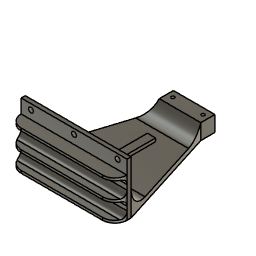
Adaptador (Autodesk Fusion 360 design; units mm, degrees)
Autodesk Fusion 360 part; units mm, degrees
sketch "Esboço1" plane through (0, 0, 0) normal (0, 0, 1) x (1, 0, 0)
  line L0 (0, 0) -> (65, 0)
  line L1 (0, 0) -> (-65, 0)
  line L2 (-65, 0) -> (-65, 5)
  line L3 (65, 0) -> (65, 5)
  line L4 (-65, 5) -> (65, 5)
  constraint coincident L0.start L1.start
  constraint horizontal L0
  constraint parallel L0 L1
  constraint perpendicular L1 L2
  constraint perpendicular L0 L3
  constraint perpendicular L3 L4
extrude "Extrusão1" add sketch "Esboço1" along normal blind 65 makes body 1
sketch "Esboço2" plane through (0, 0, 0) normal (0, 1, 0) x (1, 0, 0)
  line L0 (-65, 0) -> (-65, -15)
  line L1 (-65, -15) -> (65, -15)
  line L2 (65, -15) -> (65, 0)
  dimension "d7" = 15
  constraint vertical L0
  constraint perpendicular L0 L1
  constraint perpendicular L1 L2
  measures "d7" distance of L0.start L0.end
sketch "Esboço3" plane through (0, 0, 0) normal (0, 0, 1) x (1, 0, 0)
  line L0 (0.0189, 130) -> (-25.4811, 130)
  line L1 (0.0189, 130) -> (25.5189, 130)
  line L2 (-25.4811, 130) -> (-65, 5)
  line L3 (25.5189, 130) -> (65, 5)
  line L4 (65, 5) -> (-65, 5)
  line L5 (0, 0) -> (0, 130)
  dimension "d68" = 130
  constraint horizontal L4
  constraint coincident L5.start origin
  constraint perpendicular L4 L5
  measures "d68" distance of L5.start L5.end
extrude "Extrusão2" add sketch "Esboço3" along normal blind 6 bodies 1
sketch "Esboço4" plane through (0, 0, 0) normal (0, 0, 1) x (1, 0, 0)
  line L0 (-25.4811, 130) -> (-25.4811, 137.353)
  line L1 (25.5189, 130) -> (25.5189, 137.353)
  line L2 (25.5189, 137.353) -> (-25.4811, 137.353)
  line L3 (-25.4811, 130) -> (25.5189, 130)
  point P0 (25.5189, 130)
  constraint vertical L0
  constraint vertical L1
  constraint perpendicular L1 L2
  constraint coincident P0 L1.start
extrude "Extrusão4" add sketch "Esboço4" against normal blind 9 separate body makes body 2
extrude "Extrusão5" add sketch "Esboço4" along normal blind 6 bodies 1 2
sketch "Esboço5" plane through (0, 0, 0) normal (0, 0, 1) x (1, 0, 0)
  line L0 (0, 15) -> (-5, 15)
  line L1 (0, 15) -> (5, 15)
  line L2 (5, 15) -> (5, 95)
  line L3 (5, 95) -> (-5, 95)
  line L4 (-5, 95) -> (-5, 15)
  constraint horizontal L0
  constraint parallel L0 L1
  constraint perpendicular L1 L2
  constraint perpendicular L2 L3
  constraint perpendicular L0 L4
extrude "Extrusão6" add sketch "Esboço5" along normal blind 10 bodies 1
sketch "Esboço6" plane through (0, 0, 0) normal (0, 1, 0) x (1, 0, 0)
extrude "Extrusão7" add 1 faces at (-8.4811, 132.451, -9) along direction (0, 0, -1) blind 7 on bodies 1 bodies 1
extrude "Extrusão8" add 1 faces at (-8.4811, 137.353, -8.6667) along direction (0, 1, 0) blind 10 on bodies 1 bodies 1
sketch "Esboço7" plane through (0, 0, 0) normal (0, -1, 0) x (1, 0, 0)
  line L0 (-65, 0) -> (65, 0)
  line L1 (65, 0) -> (65, 65)
  line L2 (65, 65) -> (-65, 65)
  line L3 (-65, 65) -> (-65, 0)
  line L4 (-65, 48) -> (65, 48)
  line L5 (-65, 48) -> (65, 48)
  line L6 (65, 48) -> (65, 45)
  line L7 (65, 45) -> (-65, 45)
  line L8 (-65, 45) -> (-65, 48)
  line L9 (-65, 25) -> (65, 25)
  line L10 (65, 25) -> (65, 22)
  line L11 (65, 22) -> (-65, 22)
  line L12 (-65, 22) -> (-65, 25)
  line L13 (-65, 0) -> (65, 0)
  line L14 (65, 0) -> (65, 3)
  line L15 (65, 3) -> (-65, 3)
  line L16 (-65, 3) -> (-65, 0)
  dimension "d69" = 17
  dimension "d70" = 3
  dimension "d71" = 3
  dimension "d72" = 3
  dimension "d75" = 19
  constraint coincident L3 L4.start
  constraint coincident L1 L4.end
  constraint perpendicular L1 L4
  constraint horizontal L5
  constraint vertical L6
  constraint horizontal L7
  constraint vertical L8
  constraint horizontal L9
  constraint vertical L10
  constraint horizontal L11
  constraint vertical L12
  constraint coincident L3 L9.start
  constraint horizontal L13
  constraint vertical L14
  constraint horizontal L15
  constraint vertical L16
  constraint coincident L0.start L3.end
  measures "d69" distance of L2 L4
  measures "d70" distance of L4.start L7.end
  measures "d71" distance of L9.start L11.end
  measures "d72" distance of L0.start L15.end
  measures "d75" distance of L11 L15
hole "Furo6" at (-0.0241, 0, 58.8054) direction (0, 1, 0) diameter 6 depth 30 tip angle 118 bodies 1
hole "Furo7" at (-52.9048, 0, 58.2429) direction (0, 1, 0) diameter 6 depth 30 tip angle 118 bodies 1
hole "Furo8" at (53.4557, 0, 59.0312) direction (0, 1, 0) diameter 6 depth 30 tip angle 118 bodies 1
sketch "Esboço8" plane through (0, 0, 6) normal (0, 0, 1) x (-1, 0, 0)
  line L0 (-25.5189, -130) -> (-25.5189, -147.353)
  line L1 (-25.5189, -147.353) -> (25.4811, -147.353)
  line L2 (25.4811, -147.353) -> (25.4811, -130)
  line L3 (25.4811, -130) -> (-25.5189, -130)
  line L4 (-25.5189, -147.353) -> (25.4811, -147.353)
  line L5 (5, -15) -> (5, -95)
  line L6 (5, -95) -> (-5, -95)
  line L7 (-5, -95) -> (-5, -15)
  line L8 (-5, -15) -> (5, -15)
  line L9 (25.4811, -130) -> (65, -5)
  line L10 (65, -5) -> (-65, -5)
  line L11 (-65, -5) -> (-25.5189, -130)
  constraint coincident L2.end L3.start
  constraint coincident L0.start L3.end
  constraint coincident L0.end L1.start
  constraint coincident L1.end L2.start
extrude "Extrusão9" add sketch "Esboço8" along normal blind 13 contours L0 L1 L2 L3 L4 bodies 1
sketch "Esboço9" plane through (0, 0, 0) normal (0, 0, 1) x (1, 0, 0)
hole "Furo9" at (-18.4811, 139.853, 19) direction (0, 0, -1) diameter 4 depth 50 tip angle 118 bodies 1
hole "Furo10" at (18.5189, 139.853, 19) direction (0, 0, -1) diameter 4 depth 50 tip angle 118 bodies 1
extrude "Extrusão10" cut 1 faces at (5.8101, 132.7335, -16) along direction (0, 0, 1) blind 20 on bodies 1 bodies 1
extrude "Extrusão11" add 1 faces at (5.8101, 132.7335, 4) along direction (0, 0, -1) blind 4 on bodies 1 bodies 1
fillet "Arredondamento1" radius 25 2 edges at (0.0189, 130, 6) (0, 5, 6) on bodies 1
extrude "Extrusão12" add sketch "Esboço7" along normal blind 15 contours L0 L1 L3 L13 L14 L15 L16 | L1 L3 L9 L10 L11 L12 | L1 L3 L4 L5 L6 L7 L8 bodies 1
fillet "Arredondamento2" radius 7 4 edges at (0, 0, 3) (0, 0, 22) (0, 0, 25) (0, 0, 45) on bodies 1
fillet "Arredondamento2" radius 15 6 edges at (65, -15, 46.5) (65, -15, 23.5) (65, -15, 1.5) (-65, -15, 1.5) (-65, -15, 23.5) (-65, -15, 46.5) on bodies 1
equation "d71 = d70"
equation "d72 = d70"
